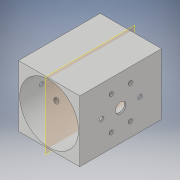
# Autodesk Inventor part: AlumConnectorForArm
Saved by Autodesk Inventor 2018.2 (Build 222227000, 227)
## iProperties
Created: 2018-01-07
Part Number: AlumConnectorForArm
Material: Generic
Document SubType Name: Modeling
Designer: steele
Density: 1 g/cm^3
Appearance: Default
Author: steele
Autodesk Inventor part; units mm, degrees
ref_plane "XZ Plane" through (0, 0, 0) normal (0, 1, 0) x (-1, 0, 0)
ref_plane "XY Plane" through (0, 0, 0) normal (0, 0, 1) x (1, 0, 0)
sketch "Sketch1" plane through (0, 0, 0) normal (0, 0, 1) x (1, 0, 0)
  line L0 (-38.1, -38.1) -> (38.1, -38.1)
  line L1 (38.1, -38.1) -> (38.1, 38.1)
  line L2 (38.1, 38.1) -> (-38.1, 38.1)
  line L3 (-38.1, 38.1) -> (-38.1, -38.1)
  line L4 (-38.1, -38.1) -> (38.1, 38.1) construction
  line L5 (38.1, -38.1) -> (-38.1, 38.1) construction
  circle A0 centre (0, 0) radius 36.5125
  dimension "d0" = 76.2
  dimension "d1" = 76.2
  dimension "d2" = 73.025
  constraints: 12 end point, 2 midpoint, 2 parallel, 1 centre point, 1 coincident, 1 horizontal, 1 perpendicular
  measures "d0" distance of L0.start L0.end
  measures "d1" distance of L1.end L0.end
  measures "d2" diameter of A0
extrude "Extrusion1" add sketch "Sketch1" against normal blind 101.6
sketch "Sketch2" plane through (38.1, -38.1, 0) normal (1, 0, 0) x (0, 0, -1)
  circle A0 centre (50.8, 38.1) radius 23.8125 construction
  line L0 (0, 0) -> (0, 76.2) construction
  point P0 (0, 38.1)
  point P1 (26.9875, 38.1)
  point P2 (38.8937, 58.7222)
  point P3 (62.7062, 58.7222)
  point P4 (74.6125, 38.1)
  point P5 (62.7063, 17.4778)
  point P6 (38.8938, 17.4778)
  dimension "d5" = 47.625
  dimension "d6" = 50.8
  dimension "d9" = 360
  constraints: 2 coincident, 1 horizontal alignment, 12 other
  measures "d6" distance from line of point (50.8, 38.1) L0
hole "Hole1" at (38.1, 0, -26.9875) at (38.1, 20.6222, -38.8937) at (38.1, 20.6222, -62.7062) at (38.1, 0, -74.6125) at (38.1, -20.6222, -62.7063) at (38.1, -20.6222, -38.8938) direction (-1, 0, 0) diameter 5.1054 end through all clearance for "Flat Head Machine Screw (82)" size "#10" standard "Ansi Unified Screw Threads"
sketch "Sketch3" plane through (38.1, -38.1, 0) normal (1, 0, 0) x (0, 0, -1)
  circle A0 centre (50.8, 38.1) radius 6.35
  line L0 (0, 0) -> (0, 76.2) projected
  point P0 (0, 38.1)
  dimension "d18" = 50.8
  dimension "d19" = 12.7
  constraints: 1 centre point
  measures "d18" distance from line of A0.centre L0
  measures "d19" diameter of A0
extrude "Extrusion2" cut sketch "Sketch3" against normal through all
body "Solid1"
